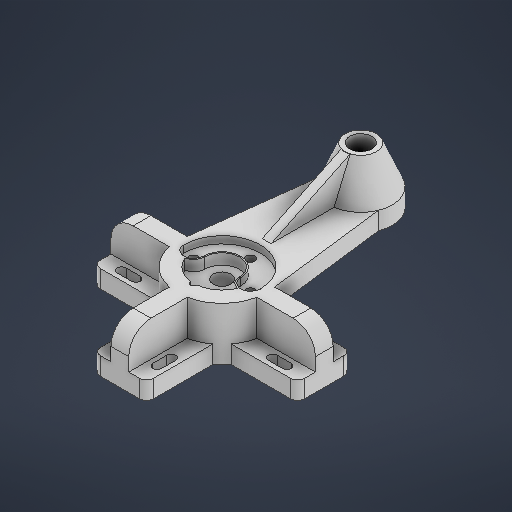
# Autodesk Inventor part: b4
Saved by Autodesk Inventor 2025.4 (Build 294407000, 407)
## iProperties
Created: 2026-05-18
Part Number: b4
Material: Generic
Document SubType Name: Modeling
Designer: VuQuan
Density: 1 g/cm^3
Appearance: Default
Author: VuQuan
Autodesk Inventor part; units mm, degrees
ref_plane "YZ Plane" through (0, 0, 0) normal (1, 0, 0) x (0, 1, 0)
ref_plane "XZ Plane" through (0, 0, 0) normal (0, 1, 0) x (-1, 0, 0)
ref_plane "XY Plane" through (0, 0, 0) normal (0, 0, 1) x (1, 0, 0)
sketch "Sketch1" plane through (0, 0, 0) normal (0, 1, 0) x (-1, 0, 0)
  circle A0 centre (0, 0) radius 50.2172
  line L0 (40.2712, -30) -> (107, -30)
  line L1 (115, -22) -> (115, 22)
  line L2 (107, 30) -> (40.2712, 30)
  arc A1 (107, -30) -> (115, -22) centre (107, -22) ccw
  arc A2 (115, 22) -> (107, 30) centre (107, 22) ccw
  line L3 (93, 20) -> (77, 20) construction
  line L4 (93, 25) -> (77, 25)
  line L5 (77, 15) -> (93, 15)
  arc A3 (93, 15) -> (93, 25) centre (93, 20) ccw
  arc A4 (77, 25) -> (77, 15) centre (77, 20) ccw
  line L6 (115, 0) -> (-115, 0) construction
  line L7 (93, -20) -> (77, -20) construction
  line L8 (93, -25) -> (77, -25)
  line L9 (77, -15) -> (93, -15)
  arc A5 (93, -25) -> (93, -15) centre (93, -20) ccw
  arc A6 (77, -15) -> (77, -25) centre (77, -20) ccw
  line L10 (115, -10) -> (49.2114, -10)
  line L11 (115, 10) -> (49.2114, 10)
  line L12 (-20, 93) -> (-20, 77) construction
  line L13 (-15, 77) -> (-15, 93)
  arc A7 (-15, 93) -> (-25, 93) centre (-20, 93) ccw
  line L14 (-10, 115) -> (-10, 49.2114)
  line L15 (22, 115) -> (-22, 115)
  line L16 (10, 115) -> (10, 49.2114)
  line L17 (-30, 107) -> (-30, 40.2712)
  line L18 (30, 40.2712) -> (30, 107)
  arc A8 (-25, 77) -> (-15, 77) centre (-20, 77) ccw
  arc A9 (30, 107) -> (22, 115) centre (22, 107) ccw
  line L19 (15, 77) -> (15, 93)
  line L20 (20, 93) -> (20, 77) construction
  arc A10 (15, 77) -> (25, 77) centre (20, 77) ccw
  line L21 (25, 93) -> (25, 77)
  arc A11 (25, 93) -> (15, 93) centre (20, 93) ccw
  line L22 (-25, 93) -> (-25, 77)
  arc A12 (-22, 115) -> (-30, 107) centre (-22, 107) ccw
  line L23 (-93, -20) -> (-77, -20) construction
  line L24 (-77, -15) -> (-93, -15)
  arc A13 (-93, -15) -> (-93, -25) centre (-93, -20) ccw
  line L25 (-115, -10) -> (-49.2114, -10)
  line L26 (-115, 22) -> (-115, -22)
  line L27 (-115, 10) -> (-49.2114, 10)
  line L28 (-107, -30) -> (-40.2712, -30)
  line L29 (-40.2712, 30) -> (-107, 30)
  arc A14 (-77, -25) -> (-77, -15) centre (-77, -20) ccw
  arc A15 (-107, 30) -> (-115, 22) centre (-107, 22) ccw
  line L30 (-77, 15) -> (-93, 15)
  line L31 (-93, 20) -> (-77, 20) construction
  arc A16 (-77, 15) -> (-77, 25) centre (-77, 20) ccw
  line L32 (-93, 25) -> (-77, 25)
  arc A17 (-93, 25) -> (-93, 15) centre (-93, 20) ccw
  line L33 (-93, -25) -> (-77, -25)
  arc A18 (-115, -22) -> (-107, -30) centre (-107, -22) ccw
  circle A19 centre (0, 0) radius 10
  point P0 (85, 20)
  point P1 (98, 20)
  point P2 (72, 20)
  point P3 (85, -20)
  point P4 (98, -20)
  point P5 (72, -20)
  point P6 (-20, 98)
  point P7 (-20, 85)
  point P8 (-20, 72)
  point P9 (0, 115)
  point P10 (20, 72)
  point P11 (20, 85)
  point P12 (20, 98)
  point P13 (-98, -20)
  point P14 (-85, -20)
  point P15 (-72, -20)
  point P16 (-115, 0)
  point P17 (-72, 20)
  point P18 (-85, 20)
  point P19 (-98, 20)
  dimension "d0" = 8
  dimension "d1" = 60
  dimension "d2" = 22
  dimension "d3" = 5
  dimension "d4" = 16
  dimension "d5" = 26
  dimension "d6" = 20
  dimension "d9" = 180
  dimension "d11" = 115
  dimension "d17" = 20
  constraints: 80 end point, 41 point on circle, 20 centre point, 11 symmetric about line, 8 tangent, 4 horizontal, 3 coincident, 3 midpoint, 3 point on line, 2 parallel, 2 perpendicular, 1 equal radius, 99 other
  measures "d0" radius of A1
  measures "d1" distance between parallel lines of L0 L2
  measures "d2" distance from line of L1 L3.start
  measures "d3" distance between parallel lines of L2 L4
  measures "d4" distance of L3.start L3.end
  measures "d5" distance of point (98, 20) point (72, 20)
  measures "d6" distance between parallel lines of L0 L10
  measures "d11" distance from line of L1 A0.centre
  measures "d17" diameter of A19
extrude "Extrusion1" add sketch "Sketch1" along normal blind 60 contours A0 | A0 L11 L1 L10 | A0 L14 L15 L16 | L25 L26 L27 A0
extrude "Extrusion2" add sketch "Sketch1" along normal blind 20 contours A0 L2 A2 L1 L11 | L10 L1 A1 L0 A0 | A0 L16 L15 A9 L18 | L28 A18 L26 L25 A0 | A0 L17 A12 L15 L14 | L27 L26 A15 L29 A0
fillet "Fillet1" radius 25 3 edges at (-115, 60, 0) (0, 60, 115) (115, 60, 0)
sketch "Sketch2" plane through (0, 60, 0) normal (0, 1, 0) x (1, 0, 0)
  circle A0 centre (0, 0) radius 10 projected
  arc A1 (10, -49.2114) -> (49.2114, -10) centre (0, 0) ccw projected
  circle A2 centre (0, -32) radius 3.75
  arc A3 (-29.5586, -12.2593) -> (-3.7436, -31.7803) centre (0, 0) ccw
  arc A4 (3.7436, -31.7803) -> (29.5586, -12.2593) centre (0, 0) ccw
  line L0 (0, -32) -> (0, 32) construction
  arc A5 (32, 0) -> (-32, 0) centre (0, 0) ccw construction
  arc A6 (43, 0) -> (-43, 0) centre (0, 0) ccw
  arc A7 (21, 0) -> (-21, 0) centre (0, 0) ccw
  arc A8 (21, 0) -> (43, 0) centre (32, 0) ccw
  arc A9 (-43, 0) -> (-21, 0) centre (-32, 0) ccw
  line L1 (-32, 0) -> (32, 0) construction
  arc A10 (-29.5586, -12.2593) -> (-19.5, 0) centre (-32, 0) ccw
  arc A11 (19.5, 0) -> (-19.5, 0) centre (0, 0) ccw
  arc A12 (19.5, 0) -> (29.5586, -12.2593) centre (32, 0) ccw
  dimension "d19" = 7.5
  dimension "d20" = 32
  dimension "d21" = 22
  dimension "d22" = 43
  dimension "d23" = 1.5
  constraints: 25 point on circle, 11 centre point, 6 coincident, 5 tangent, 4 end point, 2 midpoint, 1 horizontal, 1 horizontal alignment, 1 symmetric about line, 1 vertical, 1 other
  measures "d19" diameter of A2
  measures "d20" radius of A4
  measures "d21" radial gap between concentric circles of A6 A7
  measures "d22" radius of A6
  measures "d23" radial gap between concentric circles of A9 A10
hole "Hole2" at (32, 60, 0) at (0, 60, -32) at (-32, 60, 0) direction (0, -1, 0) diameter 10.106 depth 33 tip angle 118 counterbore diameter 13 counterbore depth 8 thread size "M12x1.75" class "6H" standard "ISO Metric profile"
extrude "Extrusion3" cut sketch "Sketch2" against normal through all contours A2
extrude "Extrusion4" cut sketch "Sketch2" against normal blind 12 contours A2 A3 A10 A11 A12 A4
extrude "Extrusion5" cut sketch "Sketch2" against normal up to surface (8 mm away) contours A8 A7 A9 A6
sketch "Sketch3" plane through (0, 60, 0) normal (0, 1, 0) x (1, 0, 0)
  arc A0 (49.2114, 10) -> (-49.2114, 10) centre (0, 0) ccw projected
  line L0 (-49.2114, 10) -> (-31.2649, 156.0588)
  line L1 (31.2649, 156.0588) -> (49.2114, 10)
  circle A1 centre (0, 152.2172) radius 31.5
  point P0 (0, 50.2172)
  dimension "d46" = 102
  dimension "d52" = 63
  constraints: 4 end point, 3 point on circle, 2 tangent, 1 centre point, 1 coincident, 1 vertical alignment
  measures "d46" distance of point (0, 152.217) point (0, 50.217)
  measures "d52" diameter of A1
extrude "Extrusion6" add sketch "Sketch3" against normal blind 20 contours A0 L0 A1 L1
ref_plane "Work Plane1" through (0, 103, 0) normal (0, 1, 0) x (1, 0, 0)
sketch "Sketch5" plane through (0, 0, 0) normal (1, 0, 0) x (0, 1, 0)
  line L0 (40, -156.0588) -> (40, -120.7172) projected
  line L1 (40, -156.0588) -> (103, -156.0588) construction
  line L2 (60, -120.7172) -> (60, -156.0588) projected
  line L3 (60, -120.7172) -> (103, -138.5588)
  line L4 (103, -138.5588) -> (103, -143.5588)
  line L5 (103, -143.5588) -> (40, -133.5588)
  line L6 (40, -120.7172) -> (60, -120.7172) projected
  line L7 (0, -50.2172) -> (40, -50.2172) projected
  line L8 (60, -50.2172) -> (60, -10) projected
  line L9 (60, -10) -> (60, -156.0588) projected
  line L10 (103, -139.3194) -> (60, -50.2172)
  point P0 (0, 0)
  point P1 (0, 0)
  point P2 (0, 0)
  dimension "d56" = 43
  dimension "d58" = 25
  dimension "d59" = 45
  dimension "d61" = 35
  constraints: 10 end point, 5 point on line, 1 horizontal, 1 parallel, 3 other
  measures "d56" distance between parallel lines of L4 L2
  measures "d58" diameter of L4.end L1
  measures "d59" diameter of L5.end L1
  measures "d61" diameter of L3.end L1
revolve "Revolution1" add sketch "Sketch5" angle 360 about axis through (0, 40, -156.0588) along (0, 1, 0) contours L0 L6 L2 L5 | L2 L3 L10 L4 L5 | L3 L4 L10
extrude "Rib1" add sketch "Sketch5" along normal mid plane 10 rib yes fills toward (81.455, -94.79) open curves L10
body "Solid1"
